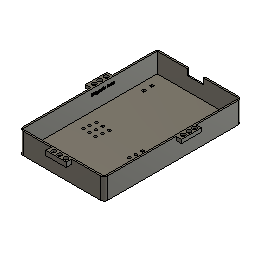
robot base (Autodesk Fusion 360 design; units mm, degrees)
Autodesk Fusion 360 part; units mm, degrees
(part 1 of 7)
sketch "Sketch1" plane through (0, 0, 0) normal (0, 1, 0) x (1, 0, 0)
  line L0 (-25, 75) -> (125, 75)
  line L1 (125, 75) -> (125, -175)
  line L2 (125, -175) -> (-25, -175)
  line L3 (-25, -175) -> (-25, 75)
  dimension "d1" = 150
  dimension "d2" = 250
  constraint horizontal L0
  constraint vertical L1
  constraint horizontal L2
  constraint vertical L3
  measures "d1" distance of L0.start L0.end
  measures "d2" distance of L0.start L2.end
extrude "Extrude1" add sketch "Sketch1" along normal blind 3 makes body 1
sketch "Sketch2" plane through (0, 3, 0) normal (0, 1, 0) x (-1, 0, 0)
  line L0 (25, 175) -> (-125, 175)
  line L1 (-125, 175) -> (-125, -75)
  line L2 (-125, -75) -> (25, -75)
  line L3 (25, -75) -> (25, 175)
sketch "Sketch3" plane through (0, 0, 0) normal (0, 1, 0) x (1, 0, 0)
  line L0 (-30, 80) -> (130, 80)
  line L1 (130, 80) -> (130, -180)
  line L2 (130, -180) -> (-30, -180)
  line L3 (-30, -180) -> (-30, 80)
  line L4 (-25, 75) -> (-25, -175)
  line L5 (125, -175) -> (125, 75)
  line L6 (125, 75) -> (-25, 75)
  dimension "d5" = 5
  dimension "d6" = 5
  dimension "d7" = 5
  constraint horizontal L0
  constraint vertical L1
  constraint horizontal L2
  constraint vertical L3
  measures "d5" distance of L3 L4
  measures "d6" distance of L1 L5
  measures "d7" distance of L0 L6
extrude "Extrude2" add sketch "Sketch3" along normal blind 40 bodies 1
shell "Shell1" thickness 3 removed faces 1 at (23.3333, 40, 93.3333) on bodies 1
move_body "Move1" bodies 1 to x (1, 0, 0) y (0, 1, 0) z (0, 0, 1) at (0, 60, 0)
sketch "Sketch4" plane through (0, 63, 0) normal (0, 1, 0) x (-1, 0, 0)
  line L0 (27, 177) -> (-127, 177)
  line L1 (-127, 177) -> (-127, -77)
  line L2 (-127, -77) -> (27, -77)
  line L3 (27, -77) -> (27, 177)
  line L4 (14.9226, -39.638) -> (9.9226, -39.638)
  line L5 (9.9226, -39.638) -> (9.9226, -34.638)
  line L6 (9.9226, -34.638) -> (14.9226, -34.638)
  line L7 (14.9226, -34.638) -> (14.9226, -39.638)
  line L8 (12.4226, 146.4275) -> (17.4226, 146.4275)
  line L9 (17.4226, 146.4275) -> (17.4226, 151.4275)
  line L10 (17.4226, 151.4275) -> (12.4226, 151.4275)
  line L11 (12.4226, 151.4275) -> (12.4226, 146.4275)
  line L12 (-110.5201, -34.638) -> (-105.5201, -34.638)
  line L13 (-105.5201, -34.638) -> (-105.5201, -39.638)
  line L14 (-105.5201, -39.638) -> (-110.5201, -39.638)
  line L15 (-110.5201, -39.638) -> (-110.5201, -34.638)
  line L16 (-105.5201, 145.9612) -> (-110.5201, 145.9612)
  line L17 (-110.5201, 145.9612) -> (-110.5201, 150.9612)
  line L18 (-110.5201, 150.9612) -> (-105.5201, 150.9612)
  line L19 (-105.5201, 150.9612) -> (-105.5201, 145.9612)
  dimension "d11" = 5
  dimension "d12" = 5
  dimension "d13" = 5
  dimension "d14" = 5
  dimension "d15" = 5
  dimension "d16" = 5
  dimension "d17" = 5
  dimension "d18" = 5
  constraint horizontal L4
  constraint vertical L5
  constraint horizontal L6
  constraint vertical L7
  constraint horizontal L8
  constraint vertical L9
  constraint horizontal L10
  constraint vertical L11
  constraint horizontal L12
  constraint vertical L13
  constraint horizontal L14
  constraint vertical L15
  constraint horizontal L16
  constraint vertical L17
  constraint horizontal L18
  constraint vertical L19
  measures "d11" distance of L4.start L4.end
  measures "d12" distance of L4.start L6.end
  measures "d13" distance of L8.start L8.end
  measures "d14" distance of L8.start L10.end
  measures "d15" distance of L12.start L12.end
  measures "d16" distance of L12.start L14.end
  measures "d17" distance of L16.start L16.end
  measures "d18" distance of L16.start L18.end
extrude "Extrude3" cut sketch "Sketch4" against normal blind 90 contours L4 L5 L6 L7 | L8 L9 L10 L11 | L12 L13 L14 L15 | L16 L17 L18 L19 bodies 1
sketch "Sketch5" plane through (0, 60, 0) normal (0, -1, 0) x (1, 0, 0)
  line L0 (110.5201, 150.9612) -> (110.5201, 145.9612)
  line L1 (110.5201, 145.9612) -> (105.5201, 145.9612)
  line L2 (105.5201, 145.9612) -> (105.5201, 150.9612)
  line L3 (105.5201, 150.9612) -> (110.5201, 150.9612)
  line L4 (105.5201, -39.638) -> (105.5201, -34.638)
  line L5 (105.5201, -34.638) -> (110.5201, -34.638)
  line L6 (110.5201, -34.638) -> (110.5201, -39.638)
  line L7 (110.5201, -39.638) -> (105.5201, -39.638)
  line L8 (-12.4226, 146.4275) -> (-17.4226, 146.4275)
  line L9 (-17.4226, 146.4275) -> (-17.4226, 151.4275)
  line L10 (-17.4226, 151.4275) -> (-12.4226, 151.4275)
  line L11 (-12.4226, 151.4275) -> (-12.4226, 146.4275)
  line L12 (-9.9226, -34.638) -> (-9.9226, -39.638)
  line L13 (-9.9226, -39.638) -> (-14.9226, -39.638)
  line L14 (-14.9226, -39.638) -> (-14.9226, -34.638)
  line L15 (-14.9226, -34.638) -> (-9.9226, -34.638)
  line L16 (130, 180) -> (-30, 180)
  line L17 (-30, 180) -> (-30, -80)
  line L18 (-30, -80) -> (130, -80)
  line L19 (130, -80) -> (130, 180)
  line L20 (-24.7646, 143.5608) -> (-4.7646, 143.5608)
  line L21 (-4.7646, 143.5608) -> (-4.7646, 93.5608)
  line L22 (-4.7646, 93.5608) -> (-24.7646, 93.5608)
  line L23 (-24.7646, 93.5608) -> (-24.7646, 143.5608)
  line L24 (-24.5171, 4.1257) -> (-4.5171, 4.1257)
  line L25 (-4.5171, 4.1257) -> (-4.5171, -45.8743)
  line L26 (-4.5171, -45.8743) -> (-24.5171, -45.8743)
  line L27 (-24.5171, -45.8743) -> (-24.5171, 4.1257)
  line L28 (123.4565, -45.8596) -> (103.4565, -45.8596)
  line L29 (103.4565, -45.8596) -> (103.4565, 4.1404)
  line L30 (103.4565, 4.1404) -> (123.4565, 4.1404)
  line L31 (123.4565, 4.1404) -> (123.4565, -45.8596)
  line L32 (104.6989, 143.7931) -> (124.6989, 143.7931)
  line L33 (124.6989, 143.7931) -> (124.6989, 93.7931)
  line L34 (124.6989, 93.7931) -> (104.6989, 93.7931)
  line L35 (104.6989, 93.7931) -> (104.6989, 143.7931)
  dimension "d21" = 20
  dimension "d22" = 50
  dimension "d23" = 20
  dimension "d24" = 50
  dimension "d25" = 20
  dimension "d26" = 50
  dimension "d27" = 20
  dimension "d28" = 50
  constraint horizontal L20
  constraint vertical L21
  constraint horizontal L22
  constraint vertical L23
  constraint horizontal L24
  constraint vertical L25
  constraint horizontal L26
  constraint vertical L27
  constraint horizontal L28
  constraint vertical L29
  constraint horizontal L30
  constraint vertical L31
  constraint horizontal L32
  constraint horizontal L34
  constraint vertical L35
  measures "d21" distance of L20.start L20.end
  measures "d22" distance of L20.start L22.end
  measures "d23" distance of L24.start L24.end
  measures "d24" distance of L24.start L26.end
  measures "d25" distance of L28.start L28.end
  measures "d26" distance of L28.start L30.end
  measures "d27" distance of L32.start L32.end
  measures "d28" distance of L32.start L34.end
extrude "Extrude4" add sketch "Sketch5" along normal blind 2 contours L4 L5 L6 L7 | L12 L13 L14 L15 | L20 L21 L22 L23 | L24 L25 L26 L27 | L28 L29 L30 L31 | L32 L33 L34 L35 bodies 1
sketch "Sketch6" plane through (0, 0, 0) normal (0, 1, 0) x (1, 0, 0)
  line L0 (-200, 100) -> (-40, 100)
  line L1 (-40, 100) -> (-40, -155)
  line L2 (-40, -155) -> (-200, -155)
  line L3 (-200, -155) -> (-200, 100)
  dimension "d31" = 160
  dimension "d32" = 255
  constraint horizontal L0
  constraint vertical L1
  constraint horizontal L2
  constraint vertical L3
  measures "d31" distance of L0.start L0.end
  measures "d32" distance of L0.start L2.end
sketch "Sketch7" plane through (0, 49.0351, -11.7723) normal (0, 0.97237, -0.233445) x (-1, 0, 0)
  line L0 (210, -96.898) -> (210, 166.4916)
  line L1 (210, 166.4916) -> (50, 166.4916)
  line L2 (50, 166.4916) -> (50, -96.898)
  line L3 (107.3171, 129.6816) -> (144.3171, 129.6816)
  line L4 (144.3171, 129.6816) -> (144.3171, 100.6816)
  line L5 (144.3171, 100.6816) -> (107.3171, 100.6816)
  line L6 (107.3171, 100.6816) -> (107.3171, 129.6816)
  line L7 (50, -96.898) -> (210, -96.898)
  dimension "d38" = 37
  dimension "d39" = 29
  constraint horizontal L3
  constraint vertical L4
  constraint horizontal L5
  constraint vertical L6
  measures "d38" distance of L3.start L3.end
  measures "d39" distance of L3.start L5.end
sketch "Sketch8" plane through (0, 49.0351, -11.7723) normal (0, 0.97237, -0.233445) x (-1, 0, 0)
  line L0 (144.3171, 129.6816) -> (144.3171, 100.6816)
  line L1 (144.3171, 100.6816) -> (107.3171, 100.6816)
  line L2 (107.3171, 100.6816) -> (107.3171, 129.6816)
  line L3 (107.3171, 129.6816) -> (144.3171, 129.6816)
  line L4 (210, -96.898) -> (210, 166.4916)
  line L5 (210, 166.4916) -> (50, 166.4916)
  line L6 (50, 166.4916) -> (50, -96.898)
  line L7 (50, -96.898) -> (210, -96.898)
copy_body "Body->Comp2" bodies 1 removing the originals makes body 2 in component "base"
sketch "Sketch9" plane through (0, 100, 0) normal (0, 1, 0) x (-1, 0, 0)
  line L0 (27, 177) -> (27, -77)
  line L1 (27, -77) -> (-127, -77)
  line L2 (-127, -77) -> (-127, 177)
  line L3 (-127, 177) -> (27, 177)
  line L4 (30, 180) -> (-130, 180)
  line L5 (-130, 180) -> (-130, -80)
  line L6 (-130, -80) -> (30, -80)
  line L7 (30, -80) -> (30, 180)
sketch "Sketch10" plane through (-30, 0, 0) normal (-1, 0, 0) x (0, 0, 1)
  line L0 (-80, 60) -> (180, 60)
  line L1 (180, 60) -> (180, 100)
  line L2 (180, 100) -> (-80, 100)
  line L3 (-80, 100) -> (-80, 60)
  line L4 (5, 100) -> (45, 100)
  line L5 (45, 100) -> (45, 94.0332)
  line L6 (45, 94.0332) -> (5, 94.0332)
  line L7 (5, 94.0332) -> (5, 100)
  dimension "d46" = 40
  constraint horizontal L4
  constraint vertical L5
  constraint horizontal L6
  constraint vertical L7
  constraint coincident L2 L4.start
  measures "d46" distance of L4.start L4.end
extrude "Extrude1'" add sketch "Sketch10" along normal blind 10 contours L2 L4 L5 L6 L7 bodies 2 in component "base"
sketch "Sketch11" plane through (0, 100, 0) normal (0, 1, 0) x (-1, 0, 0)
  line L0 (27, 177) -> (27, -77)
  line L1 (27, -77) -> (-127, -77)
  line L2 (-127, -77) -> (-127, 177)
  line L3 (-127, 177) -> (27, 177)
  line L4 (30, 180) -> (-130, 180)
  line L5 (-130, 180) -> (-130, -80)
  line L6 (-130, -80) -> (30, -80)
  line L7 (30, -80) -> (30, 5)
  line L8 (30, 5) -> (40, 5)
  line L9 (40, 5) -> (40, 45)
  line L10 (40, 45) -> (30, 45)
  line L11 (30, 45) -> (30, 180)
  circle A0 centre (33.1089, 35.6235) radius 4
  circle A1 centre (33.528, 24.7269) radius 4
  circle A2 centre (33.7376, 12.573) radius 4
  dimension "d49" = 8
  dimension "d50" = 8
  dimension "d51" = 8
  measures "d49" diameter of A0
  measures "d50" diameter of A1
  measures "d51" diameter of A2
extrude "Extrude2'" cut sketch "Sketch11" against normal blind 4 contours A0 | A1 | A2 bodies 2 in component "base"
sketch "Sketch12" plane through (130, 0, 0) normal (1, 0, 0) x (0, 0, -1)
  line L0 (-180, 60) -> (80, 60)
  line L1 (80, 60) -> (80, 100)
  line L2 (80, 100) -> (-180, 100)
  line L3 (-180, 100) -> (-180, 60)
  line L4 (-44.1105, 100) -> (-6.5994, 100)
  line L5 (-6.5994, 100) -> (-6.5994, 93.0994)
  line L6 (-6.5994, 93.0994) -> (-44.1105, 93.0994)
  line L7 (-44.1105, 93.0994) -> (-44.1105, 100)
  constraint horizontal L4
  constraint horizontal L6
  constraint vertical L7
  constraint coincident L2 L4.start
extrude "Extrude3'" add sketch "Sketch12" along normal blind 10 contours L2 L4 L5 L6 L7 bodies 2 in component "base"
sketch "Sketch13" plane through (0, 100, 0) normal (0, 1, 0) x (-1, 0, 0)
  circle A0 centre (33.1089, 35.6235) radius 4
  circle A1 centre (33.528, 24.7269) radius 4
  circle A2 centre (33.7376, 12.573) radius 4
  line L0 (27, 177) -> (27, -77)
  line L1 (27, -77) -> (-127, -77)
  line L2 (-127, -77) -> (-127, 177)
  line L3 (-127, 177) -> (27, 177)
  line L4 (30, 180) -> (-130, 180)
  line L5 (-130, 180) -> (-130, 44.1105)
  line L6 (-130, 44.1105) -> (-140, 44.1105)
  line L7 (-140, 44.1105) -> (-140, 6.5994)
  line L8 (-140, 6.5994) -> (-130, 6.5994)
  line L9 (-130, 6.5994) -> (-130, -80)
  line L10 (-130, -80) -> (30, -80)
  line L11 (30, -80) -> (30, 5)
  line L12 (30, 5) -> (40, 5)
  line L13 (40, 5) -> (40, 45)
  line L14 (40, 45) -> (30, 45)
  line L15 (30, 45) -> (30, 180)
sketch "Sketch14" plane through (130, 0, 0) normal (1, 0, 0) x (0, 0, -1)
sketch "Sketch15" plane through (0, 100, 0) normal (0, 1, 0) x (-1, 0, 0)
  circle A0 centre (-133.6931, 13.6208) radius 4
  circle A1 centre (-134, 24) radius 4
  circle A2 centre (-134, 35) radius 4
  dimension "d56" = 8
  dimension "d57" = 8
  dimension "d58" = 8
  measures "d56" diameter of A0
  measures "d57" diameter of A1
  measures "d58" diameter of A2
extrude "Extrude4'" cut sketch "Sketch15" against normal blind 4 bodies 2 in component "base"
sketch "Sketch16" plane through (131.259, 0, 0) normal (1, 0, 0) x (0, 0, -1)
  line L0 (-178.8896, 102.3306) -> (76.1007, 100.1054)
  line L1 (76.1007, 100.1054) -> (76.136, 104.1577)
  line L2 (76.136, 104.1577) -> (-178.2788, 172.328)
  line L3 (-178.2788, 172.328) -> (-178.8896, 102.3306)
  line L4 (-45, 110) -> (-6.7003, 110)
  line L5 (-6.7003, 110) -> (-6.7003, 101.218)
  line L6 (-6.7003, 101.218) -> (-45, 101.218)
  line L7 (-45, 101.218) -> (-45, 110)
  constraint horizontal L4
  constraint vertical L5
  constraint horizontal L6
  constraint vertical L7
sketch "Sketch17" plane through (0, 100, 0) normal (0, 1, 0) x (-1, 0, 0)
  circle A0 centre (-136.21, 34.8) radius 4
  circle A1 centre (-135.94, 25.4) radius 4
  circle A2 centre (-135.73, 15.73) radius 4
  dimension "d63" = 8
  dimension "d64" = 8
  dimension "d65" = 8
  measures "d63" diameter of A0
  measures "d64" diameter of A1
  measures "d65" diameter of A2
sketch "Sketch18" plane through (-29.741, 0, 0) normal (-1, 0, 0) x (0, 0, 1)
  line L0 (-76.1007, 100.1054) -> (178.8896, 102.3306)
  line L1 (178.8896, 102.3306) -> (178.2788, 172.328)
  line L2 (178.2788, 172.328) -> (-76.136, 104.1577)
  line L3 (-76.136, 104.1577) -> (-76.1007, 100.1054)
  line L4 (4.8558, 101.218) -> (45, 101.218)
  line L5 (45, 101.218) -> (45, 108)
  line L6 (45, 108) -> (4.8558, 108)
  line L7 (4.8558, 108) -> (4.8558, 101.218)
  constraint horizontal L4
  constraint vertical L5
  constraint horizontal L6
  constraint vertical L7
sketch "Sketch19" plane through (0, 101.218, 0) normal (0, -1, 0) x (1, 0, 0)
  line L0 (-29.741, 4.8558) -> (-29.741, 45)
  line L1 (-29.741, 45) -> (-39.741, 45)
  line L2 (-39.741, 45) -> (-39.741, 4.8558)
  line L3 (-39.741, 4.8558) -> (-29.741, 4.8558)
  circle A0 centre (-35, 13) radius 4
  circle A1 centre (-35, 23) radius 4
  circle A2 centre (-35, 33) radius 4
  dimension "d70" = 8
  dimension "d71" = 8
  dimension "d72" = 8
  measures "d70" diameter of A0
  measures "d71" diameter of A1
  measures "d72" diameter of A2
sketch "Sketch20" plane through (0, 0, 180) normal (0, 0, 1) x (1, 0, 0)
  line L0 (-30, 60) -> (130, 60)
  line L1 (130, 60) -> (130, 100)
  line L2 (130, 100) -> (-30, 100)
  line L3 (-30, 100) -> (-30, 60)
  line L4 (30, 100) -> (68.2649, 100)
  line L5 (68.2649, 100) -> (68.2649, 91.3001)
  line L6 (68.2649, 91.3001) -> (30, 91.3001)
  line L7 (30, 91.3001) -> (30, 100)
  constraint horizontal L4
  constraint vertical L5
  constraint horizontal L6
  constraint vertical L7
  constraint coincident L2 L4.start
extrude "Extrude5" add sketch "Sketch20" along normal blind 10 contours L2 L4 L5 L6 L7 bodies 2 in component "base"
sketch "Sketch21" plane through (0, 0, 0) normal (0, 0, 1) x (1, 0, 0)
sketch "Sketch22" plane through (0, 100, 0) normal (0, 1, 0) x (-1, 0, 0)
  circle A0 centre (-134, 35) radius 4
  circle A1 centre (-134, 24) radius 4
  circle A2 centre (-133.6931, 13.6208) radius 4
  circle A3 centre (33.1089, 35.6235) radius 4
  circle A4 centre (33.528, 24.7269) radius 4
  circle A5 centre (33.7376, 12.573) radius 4
  line L0 (27, 177) -> (27, -77)
  line L1 (27, -77) -> (-127, -77)
  line L2 (-127, -77) -> (-127, 177)
  line L3 (-127, 177) -> (27, 177)
  line L4 (30, 180) -> (-30, 180)
  line L5 (-30, 180) -> (-30, 190)
  line L6 (-30, 190) -> (-68.2649, 190)
  line L7 (-68.2649, 190) -> (-68.2649, 180)
  line L8 (-68.2649, 180) -> (-130, 180)
  line L9 (-130, 180) -> (-130, 44.1105)
  line L10 (-130, 44.1105) -> (-140, 44.1105)
  line L11 (-140, 44.1105) -> (-140, 6.5994)
  line L12 (-140, 6.5994) -> (-130, 6.5994)
  line L13 (-130, 6.5994) -> (-130, -80)
  line L14 (-130, -80) -> (30, -80)
  line L15 (30, -80) -> (30, 5)
  line L16 (30, 5) -> (40, 5)
  line L17 (40, 5) -> (40, 45)
  line L18 (40, 45) -> (30, 45)
  line L19 (30, 45) -> (30, 180)
  circle A6 centre (-39, 184) radius 4
  circle A7 centre (-50, 184) radius 4
  circle A8 centre (-62, 184) radius 4
  dimension "d77" = 8
  dimension "d78" = 8
  dimension "d79" = 8
  measures "d77" diameter of A6
  measures "d78" diameter of A7
  measures "d79" diameter of A8
extrude "Extrude6" cut sketch "Sketch22" against normal blind 4 contours A6 | A7 | A8 bodies 2 in component "base"
sketch "Sketch23" plane through (0, 1.5688, 179.7689) normal (0, 0.008727, 0.999962) x (1, 0, 0)
  line L0 (-29.741, 100.7657) -> (130.259, 100.7657)
  line L1 (130.259, 100.7657) -> (130.259, 170.7657)
  line L2 (130.259, 170.7657) -> (-29.741, 170.7657)
  line L3 (-29.741, 170.7657) -> (-29.741, 100.7657)
  line L4 (30, 109) -> (68.1162, 109)
  line L5 (68.1162, 109) -> (68.1162, 100.7657)
  line L6 (68.1162, 100.7657) -> (30, 100.7657)
  line L7 (30, 100.7657) -> (30, 109)
  constraint horizontal L4
  constraint horizontal L6
  constraint vertical L7
  constraint coincident L0 L5.end
sketch "Sketch24" plane through (0, 100.7618, -0.8793) normal (0, -0.999962, 0.008727) x (1, 0, 0)
  line L0 (127.259, 176.7758) -> (127.259, -72.2242)
  line L1 (127.259, -72.2242) -> (-26.741, -72.2242)
  line L2 (-26.741, -72.2242) -> (-26.741, 176.7758)
  line L3 (-26.741, 176.7758) -> (127.259, 176.7758)
  line L4 (-29.741, -75.2242) -> (130.259, -75.2242)
  line L5 (130.259, -75.2242) -> (130.259, 179.7758)
  line L6 (130.259, 179.7758) -> (68.1162, 179.7758)
  line L7 (68.1162, 179.7758) -> (68.1162, 190.7758)
  line L8 (68.1162, 190.7758) -> (30, 190.7758)
  line L9 (30, 190.7758) -> (30, 179.7758)
  line L10 (30, 179.7758) -> (-29.741, 179.7758)
  line L11 (-29.741, 179.7758) -> (-29.741, -75.2242)
  circle A0 centre (39.3165, 184.6097) radius 4
  circle A1 centre (50, 185) radius 4
  circle A2 centre (60, 185) radius 4
  dimension "d84" = 8
  dimension "d85" = 8
  dimension "d86" = 8
  measures "d84" diameter of A0
  measures "d85" diameter of A1
  measures "d86" diameter of A2
sketch "Sketch25" plane through (0, 1.5688, 179.7689) normal (0, 0.008727, 0.999962) x (1, 0, 0)
  line L0 (68.1162, 109) -> (68.1162, 100.7657)
  line L1 (68.1162, 100.7657) -> (130.259, 100.7657)
  line L2 (130.259, 100.7657) -> (130.259, 170.7657)
  line L3 (130.259, 170.7657) -> (-29.741, 170.7657)
  line L4 (-29.741, 170.7657) -> (-29.741, 100.7657)
  line L5 (-29.741, 100.7657) -> (30, 100.7657)
  line L6 (30, 100.7657) -> (30, 109)
  line L7 (30, 109) -> (68.1162, 109)
  line L8 (5, 145) -> (10, 145)
  line L9 (10, 145) -> (10, 135)
  line L10 (10, 135) -> (5, 135)
  line L11 (5, 135) -> (5, 145)
  line L12 (15, 145) -> (20, 145)
  line L13 (20, 145) -> (20, 135)
  line L14 (20, 135) -> (15, 135)
  line L15 (15, 135) -> (15, 145)
  line L16 (25, 145) -> (30, 145)
  line L17 (30, 145) -> (30, 135)
  line L18 (30, 135) -> (25, 135)
  line L19 (25, 135) -> (25, 145)
  line L20 (35, 145) -> (40, 145)
  line L21 (40, 145) -> (40, 135)
  line L22 (40, 135) -> (35, 135)
  line L23 (35, 135) -> (35, 145)
  line L24 (45, 145) -> (50, 145)
  line L25 (50, 145) -> (50, 135)
  line L26 (50, 135) -> (45, 135)
  line L27 (45, 135) -> (45, 145)
  line L28 (55, 145) -> (60, 145)
  line L29 (60, 145) -> (60, 135)
  line L30 (60, 135) -> (55, 135)
  line L31 (55, 135) -> (55, 145)
  line L32 (65, 145) -> (70, 145)
  line L33 (70, 145) -> (70, 135)
  line L34 (70, 135) -> (65, 135)
  line L35 (65, 135) -> (65, 145)
  line L36 (75, 145) -> (80, 145)
  line L37 (80, 145) -> (80, 135)
  line L38 (80, 135) -> (75, 135)
  line L39 (75, 135) -> (75, 145)
  line L40 (85, 145) -> (90, 145)
  line L41 (90, 145) -> (90, 135)
  line L42 (90, 135) -> (85, 135)
  line L43 (85, 135) -> (85, 145)
  line L44 (95, 145) -> (100, 145)
  line L45 (100, 145) -> (100, 135)
  line L46 (100, 135) -> (95, 135)
  line L47 (95, 135) -> (95, 145)
  line L48 (5, 125) -> (10, 125)
  line L49 (10, 125) -> (10, 115)
  line L50 (10, 115) -> (5, 115)
  line L51 (5, 115) -> (5, 125)
  line L52 (15, 125) -> (20, 125)
  line L53 (20, 125) -> (20, 115)
  line L54 (20, 115) -> (15, 115)
  line L55 (15, 115) -> (15, 125)
  line L56 (25, 125) -> (30, 125)
  line L57 (30, 125) -> (30, 115)
  line L58 (30, 115) -> (25, 115)
  line L59 (25, 115) -> (25, 125)
  line L60 (35, 125) -> (40, 125)
  line L61 (40, 125) -> (40, 115)
  line L62 (40, 115) -> (35, 115)
  line L63 (35, 115) -> (35, 125)
  line L64 (45, 125) -> (50, 125)
  line L65 (50, 125) -> (50, 115)
  line L66 (50, 115) -> (45, 115)
  line L67 (45, 115) -> (45, 125)
  line L68 (55, 125) -> (60, 125)
  line L69 (60, 125) -> (60, 115)
  line L70 (60, 115) -> (55, 115)
  line L71 (55, 115) -> (55, 125)
  line L72 (65, 125) -> (70, 125)
  line L73 (70, 125) -> (70, 115)
  line L74 (70, 115) -> (65, 115)
  line L75 (65, 115) -> (65, 125)
  line L76 (75, 125) -> (80, 125)
  line L77 (80, 125) -> (80, 115)
  line L78 (80, 115) -> (75, 115)
  line L79 (75, 115) -> (75, 125)
  line L80 (85, 125) -> (90, 125)
  line L81 (90, 125) -> (90, 115)
  line L82 (90, 115) -> (85, 115)
  line L83 (85, 115) -> (85, 125)
  line L84 (95, 125) -> (100, 125)
  line L85 (100, 125) -> (100, 115)
  line L86 (100, 115) -> (95, 115)
  line L87 (95, 115) -> (95, 125)
  constraint horizontal L8
  constraint vertical L9
  constraint horizontal L10
  constraint vertical L11
  constraint horizontal L12
  constraint vertical L13
  constraint horizontal L14
  constraint vertical L15
  constraint horizontal L16
  constraint vertical L17
  constraint horizontal L18
  constraint vertical L19
  constraint horizontal L20
  constraint vertical L21
  constraint horizontal L22
  constraint vertical L23
  constraint horizontal L24
  constraint vertical L25
  constraint horizontal L26
  constraint vertical L27
  constraint horizontal L28
  constraint vertical L29
  constraint horizontal L30
  constraint vertical L31
  constraint horizontal L32
  constraint vertical L33
  constraint horizontal L34
  constraint vertical L35
  constraint horizontal L36
  constraint vertical L37
  constraint horizontal L38
  constraint vertical L39
  constraint horizontal L40
  constraint vertical L41
  constraint horizontal L42
  constraint vertical L43
  constraint horizontal L44
  constraint vertical L45
  constraint horizontal L46
  constraint vertical L47
  constraint horizontal L48
  constraint vertical L49
  constraint horizontal L50
  constraint vertical L51
  constraint horizontal L52
  constraint vertical L53
  constraint horizontal L54
  constraint vertical L55
  constraint horizontal L56
  constraint vertical L57
  constraint horizontal L58
  constraint vertical L59
  constraint horizontal L60
  constraint vertical L61
  constraint horizontal L62
  constraint vertical L63
  constraint horizontal L64
  constraint vertical L65
  constraint horizontal L66
  constraint vertical L67
  constraint horizontal L68
  constraint vertical L69
  constraint horizontal L70
  constraint vertical L71
  constraint horizontal L72
  constraint vertical L73
  constraint horizontal L74
  constraint vertical L75
  constraint horizontal L76
  constraint vertical L77
  constraint horizontal L78
  constraint vertical L79
  constraint horizontal L80
  constraint vertical L81
  constraint horizontal L82
  constraint vertical L83
  constraint horizontal L84
  constraint vertical L85
  constraint horizontal L86
  constraint vertical L87
sketch "Sketch26" plane through (-29.741, 0, 0) normal (-1, 0, 0) x (0, 0, 1)
  line L0 (4.8558, 108) -> (45, 108)
  line L1 (45, 108) -> (45, 101.218)
  line L2 (45, 101.218) -> (4.8558, 101.218)
  line L3 (4.8558, 101.218) -> (4.8558, 108)
  line L4 (-76.1007, 100.1054) -> (178.8896, 102.3306)
  line L5 (178.8896, 102.3306) -> (178.2788, 172.328)
  line L6 (178.2788, 172.328) -> (-76.136, 104.1577)
  line L7 (-76.136, 104.1577) -> (-76.1007, 100.1054)
sketch "Sketch27" plane through (0, 63, 0) normal (0, 1, 0) x (-1, 0, 0)
  line L0 (-110.5201, 145.9612) -> (-110.5201, 150.9612)
  line L1 (-110.5201, 150.9612) -> (-105.5201, 150.9612)
  line L2 (-105.5201, 150.9612) -> (-105.5201, 145.9612)
  line L3 (-105.5201, 145.9612) -> (-110.5201, 145.9612)
  line L4 (-105.5201, -34.638) -> (-105.5201, -39.638)
  line L5 (-105.5201, -39.638) -> (-110.5201, -39.638)
  line L6 (-110.5201, -39.638) -> (-110.5201, -34.638)
  line L7 (-110.5201, -34.638) -> (-105.5201, -34.638)
  line L8 (17.4226, 146.4275) -> (12.4226, 146.4275)
  line L9 (12.4226, 146.4275) -> (12.4226, 151.4275)
  line L10 (12.4226, 151.4275) -> (17.4226, 151.4275)
  line L11 (17.4226, 151.4275) -> (17.4226, 146.4275)
  line L12 (9.9226, -39.638) -> (9.9226, -34.638)
  line L13 (9.9226, -34.638) -> (14.9226, -34.638)
  line L14 (14.9226, -34.638) -> (14.9226, -39.638)
  line L15 (14.9226, -39.638) -> (9.9226, -39.638)
  line L16 (27, 177) -> (-127, 177)
  line L17 (-127, 177) -> (-127, -77)
  line L18 (-127, -77) -> (27, -77)
  line L19 (27, -77) -> (27, 177)
  line L20 (-106.0146, 110.336) -> (-106.0146, 147.3829) construction
  line L21 (-106.0146, 147.3829) -> (-117.9945, 147.3829) construction
  line L22 (-117.9945, 147.3829) -> (-117.9945, 110.336) construction
  line L23 (-117.9945, 110.336) -> (-106.0146, 110.336) construction
  dimension "d91" = 6
  text T0 "Hole for\nTT wire" font "Arial" height 6 align left top in box 37.0468 x 11.9799 at (-106.0146, 110.336) x (0, 1) y (-1, 0) spacing 1 kerned
sketch "Sketch28" plane through (0, 0, 0) normal (0, 0, 1) x (1, 0, 0)
sketch "Sketch29" plane through (0, 0, 0) normal (0, 0, 1) x (1, 0, 0)
extrude "Extrude7" cut sketch "Sketch27" against normal blind 1.5 text T0 bodies 2 in component "base"
sketch "Sketch30" plane through (0, 0, 177) normal (0, 0, -1) x (-1, 0, 0)
  line L0 (-127, 63) -> (27, 63)
  line L1 (27, 63) -> (27, 100)
  line L2 (27, 100) -> (-127, 100)
  line L3 (-127, 100) -> (-127, 63)
  line L4 (-82.8733, 77.686) -> (-13.3336, 77.0675) construction
  line L5 (-13.3336, 77.0675) -> (-13.2091, 91.0673) construction
  line L6 (-13.2091, 91.0673) -> (-82.7488, 91.6857) construction
  line L7 (-82.7488, 91.6857) -> (-82.8733, 77.686) construction
  dimension "d95" = 6
  dimension "d96" = 0
  text T0 "Gethin Robot v1" font "Arial" height 6 bold align left top in box 69.5425 x 14.0003 at (-82.8733, 77.686) x (0.99996, -0.008893) y (0.008893, 0.99996) spacing 1 kerned
extrude "Extrude8" cut sketch "Sketch30" against normal blind 1.5 text T0 bodies 2 in component "base"
sketch "Sketch31" plane through (-27, 0, 0) normal (1, 0, 0) x (0, 0, -1)
  line L0 (-177, 63) -> (77, 63)
  line L1 (77, 63) -> (77, 100)
  line L2 (77, 100) -> (-177, 100)
  line L3 (-177, 100) -> (-177, 63)
  line L4 (-46.978, 84.5868) -> (2.0388, 84.3472) construction
  line L5 (2.0388, 84.3472) -> (2.0772, 92.1978) construction
  line L6 (2.0772, 92.1978) -> (-46.9396, 92.4374) construction
  line L7 (-46.9396, 92.4374) -> (-46.978, 84.5868) construction
  dimension "d99" = 5
  text T0 "Magnets here" font "Arial" height 5 bold align left top in box 49.0173 x 7.8507 at (-46.978, 84.5868) x (0.999988, -0.004888) y (0.004888, 0.999988) spacing 1 kerned
extrude "Extrude9" cut sketch "Sketch31" against normal blind 1.5 text T0 bodies 2 in component "base"
fillet "Fillet1" radius 7 2 edges at (-30, 80, 180) (130, 80, 180) on bodies 2 in component "base"
fillet "Fillet2" radius 7 1 edges at (130, 80, -80) on bodies 2 in component "base"
fillet "Fillet3" radius 7 1 edges at (-30, 80, -80) on bodies 2 in component "base"
sketch "Sketch32" plane through (0, 116.2145, -31.1396) normal (0, 0.965926, -0.258819) x (-1, 0, 0)
  ellipse E0 centre (22.741, -39.3535) end of major axis (22.741, -46.5838) minor radius 7 (22.741, -46.5838) -> (29.741, -39.3535) ccw
  line L0 (29.741, -39.3535) -> (29.741, 209.5755)
  ellipse E1 centre (22.741, 209.5755) end of major axis (22.741, 216.8058) minor radius 7 (29.741, 209.5755) -> (22.741, 216.8058) ccw
  line L1 (22.741, 216.8058) -> (-123.259, 216.8058)
  ellipse E2 centre (-123.259, 209.5755) end of major axis (-123.259, 216.8058) minor radius 7 (-123.259, 216.8058) -> (-130.259, 209.5755) ccw
  line L2 (-130.259, 209.5755) -> (-130.259, -39.3535)
  ellipse E3 centre (-123.259, -39.3535) end of major axis (-123.259, -46.5838) minor radius 7 (-130.259, -39.3535) -> (-123.259, -46.5838) ccw
  line L3 (-123.259, -46.5838) -> (22.741, -46.5838)
  line L4 (-35.9419, 179.9959) -> (-35.9419, 150.9959)
  line L5 (-35.9419, 150.9959) -> (-72.9419, 150.9959)
  line L6 (-72.9419, 150.9959) -> (-72.9419, 179.9959)
  line L7 (-72.9419, 179.9959) -> (-35.9419, 179.9959)
sketch "Sketch33" plane through (0, 116.2145, -31.1396) normal (0, 0.965926, -0.258819) x (-1, 0, 0)
  ellipse E0 centre (22.741, -39.3535) end of major axis (22.741, -46.5838) minor radius 7 (22.741, -46.5838) -> (29.741, -39.3535) ccw
  line L0 (29.741, -39.3535) -> (29.741, 209.5755)
  ellipse E1 centre (22.741, 209.5755) end of major axis (22.741, 216.8058) minor radius 7 (29.741, 209.5755) -> (22.741, 216.8058) ccw
  line L1 (22.741, 216.8058) -> (-123.259, 216.8058)
  ellipse E2 centre (-123.259, 209.5755) end of major axis (-123.259, 216.8058) minor radius 7 (-123.259, 216.8058) -> (-130.259, 209.5755) ccw
  line L2 (-130.259, 209.5755) -> (-130.259, -39.3535)
  ellipse E3 centre (-123.259, -39.3535) end of major axis (-123.259, -46.5838) minor radius 7 (-130.259, -39.3535) -> (-123.259, -46.5838) ccw
  line L3 (-123.259, -46.5838) -> (22.741, -46.5838)
  line L4 (-35.9419, 179.9959) -> (-35.9419, 150.9959)
  line L5 (-35.9419, 150.9959) -> (-72.9419, 150.9959)
  line L6 (-72.9419, 150.9959) -> (-72.9419, 179.9959)
  line L7 (-72.9419, 179.9959) -> (-35.9419, 179.9959)
sketch "Sketch34" plane through (0, 49.0351, -11.7723) normal (0, 0.97237, -0.233445) x (-1, 0, 0)
sketch "Sketch35" plane through (0, 116.2145, -31.1396) normal (0, 0.965926, -0.258819) x (-1, 0, 0)
  ellipse E0 centre (22.741, -39.3535) end of major axis (22.741, -46.5838) minor radius 7 (22.741, -46.5838) -> (29.741, -39.3535) ccw
  line L0 (29.741, -39.3535) -> (29.741, 209.5755)
  ellipse E1 centre (22.741, 209.5755) end of major axis (22.741, 216.8058) minor radius 7 (29.741, 209.5755) -> (22.741, 216.8058) ccw
  line L1 (22.741, 216.8058) -> (-123.259, 216.8058)
  ellipse E2 centre (-123.259, 209.5755) end of major axis (-123.259, 216.8058) minor radius 7 (-123.259, 216.8058) -> (-130.259, 209.5755) ccw
  line L2 (-130.259, 209.5755) -> (-130.259, -39.3535)
  ellipse E3 centre (-123.259, -39.3535) end of major axis (-123.259, -46.5838) minor radius 7 (-130.259, -39.3535) -> (-123.259, -46.5838) ccw
  line L3 (-123.259, -46.5838) -> (22.741, -46.5838)
  line L4 (-35.9419, 179.9959) -> (-35.9419, 150.9959)
  line L5 (-35.9419, 150.9959) -> (-72.9419, 150.9959)
  line L6 (-72.9419, 150.9959) -> (-72.9419, 179.9959)
  line L7 (-72.9419, 179.9959) -> (-35.9419, 179.9959)
sketch "Sketch36" plane through (0, 116.2145, -31.1396) normal (0, 0.965926, -0.258819) x (-1, 0, 0)
  ellipse E0 centre (22.741, -39.3535) end of major axis (22.741, -46.5838) minor radius 7 (22.741, -46.5838) -> (29.741, -39.3535) ccw
  line L0 (29.741, -39.3535) -> (29.741, 209.5755)
  ellipse E1 centre (22.741, 209.5755) end of major axis (22.741, 216.8058) minor radius 7 (29.741, 209.5755) -> (22.741, 216.8058) ccw
  line L1 (22.741, 216.8058) -> (-123.259, 216.8058)
  ellipse E2 centre (-123.259, 209.5755) end of major axis (-123.259, 216.8058) minor radius 7 (-123.259, 216.8058) -> (-130.259, 209.5755) ccw
  line L2 (-130.259, 209.5755) -> (-130.259, -39.3535)
  ellipse E3 centre (-123.259, -39.3535) end of major axis (-123.259, -46.5838) minor radius 7 (-130.259, -39.3535) -> (-123.259, -46.5838) ccw
  line L3 (-123.259, -46.5838) -> (22.741, -46.5838)
  line L4 (-35.9419, 179.9959) -> (-35.9419, 150.9959)
  line L5 (-35.9419, 150.9959) -> (-72.9419, 150.9959)
  line L6 (-72.9419, 150.9959) -> (-72.9419, 179.9959)
  line L7 (-72.9419, 179.9959) -> (-35.9419, 179.9959)
  line L8 (-105, 20) -> (4.5871, 20)
  line L9 (19.5871, 5) -> (19.5871, -24.3535)
  line L10 (4.5871, -39.3535) -> (-105, -39.3535)
  line L11 (-120, -24.3535) -> (-120, 5)
  arc A0 (-105, 20) -> (-120, 5) centre (-105, 5) ccw
  arc A1 (19.5871, 5) -> (4.5871, 20) centre (4.5871, 5) ccw
  arc A2 (4.5871, -39.3535) -> (19.5871, -24.3535) centre (4.5871, -24.3535) ccw
  arc A3 (-120, -24.3535) -> (-105, -39.3535) centre (-105, -24.3535) ccw
  dimension "d115" = 15
  constraint horizontal L8
  constraint vertical L9
  constraint horizontal L10
  constraint vertical L11
  constraint tangent L8 A0
  constraint tangent L11 A0
  constraint tangent L8 A1
  constraint tangent L9 A1
  constraint equal A0 A1
  constraint tangent L10 A2
  constraint tangent L9 A2
  constraint equal A0 A2
  constraint tangent L10 A3
  constraint tangent L11 A3
  constraint equal A0 A3
  measures "d115" radius of A0
sketch "Sketch37" plane through (0, 116.2145, -31.1396) normal (0, 0.965926, -0.258819) x (-1, 0, 0)
  ellipse E0 centre (22.741, -39.3535) end of major axis (22.741, -46.5838) minor radius 7 (22.741, -46.5838) -> (29.741, -39.3535) ccw
  line L0 (29.741, -39.3535) -> (29.741, 209.5755)
  ellipse E1 centre (22.741, 209.5755) end of major axis (22.741, 216.8058) minor radius 7 (29.741, 209.5755) -> (22.741, 216.8058) ccw
  line L1 (22.741, 216.8058) -> (-123.259, 216.8058)
  ellipse E2 centre (-123.259, 209.5755) end of major axis (-123.259, 216.8058) minor radius 7 (-123.259, 216.8058) -> (-130.259, 209.5755) ccw
  line L2 (-130.259, 209.5755) -> (-130.259, -39.3535)
  ellipse E3 centre (-123.259, -39.3535) end of major axis (-123.259, -46.5838) minor radius 7 (-130.259, -39.3535) -> (-123.259, -46.5838) ccw
  line L3 (-123.259, -46.5838) -> (22.741, -46.5838)
  line L4 (-35.9419, 179.9959) -> (-35.9419, 150.9959)
  line L5 (-35.9419, 150.9959) -> (-72.9419, 150.9959)
  line L6 (-72.9419, 150.9959) -> (-72.9419, 179.9959)
  line L7 (-72.9419, 179.9959) -> (-35.9419, 179.9959)
  line L8 (10, 30) -> (-10, 30)
  line L9 (-20, 40) -> (-20, 60)
  line L10 (-10, 70) -> (10, 70)
  line L11 (20, 60) -> (20, 40)
  line L12 (-40, 70) -> (-110, 70)
  line L13 (-120, 60) -> (-120, 40)
  line L14 (-110, 30) -> (-40, 30)
  line L15 (-30, 40) -> (-30, 60)
  arc A0 (-110, 70) -> (-120, 60) centre (-110, 60) ccw
  arc A1 (-30, 60) -> (-40, 70) centre (-40, 60) ccw
  arc A2 (-40, 30) -> (-30, 40) centre (-40, 40) ccw
  arc A3 (-120, 40) -> (-110, 30) centre (-110, 40) ccw
  arc A4 (-20, 40) -> (-10, 30) centre (-10, 40) ccw
  arc A5 (20, 60) -> (10, 70) centre (10, 60) ccw
  arc A6 (10, 30) -> (20, 40) centre (10, 40) ccw
  arc A7 (-10, 70) -> (-20, 60) centre (-10, 60) ccw
  dimension "d118" = 10
  constraint horizontal L8
  constraint vertical L9
  constraint horizontal L10
  constraint vertical L11
  constraint horizontal L12
  constraint vertical L13
  constraint horizontal L14
  constraint vertical L15
  constraint tangent L12 A0
  constraint tangent L13 A0
  constraint tangent L12 A1
  constraint tangent L15 A1
  constraint equal A0 A1
  constraint tangent L14 A2
  constraint tangent L15 A2
  constraint equal A0 A2
  constraint tangent L13 A3
  constraint tangent L14 A3
  constraint equal A0 A3
  constraint tangent L8 A4
  constraint tangent L9 A4
  constraint equal A0 A4
  constraint tangent L10 A5
  constraint tangent L11 A5
  constraint equal A0 A5
  constraint tangent L8 A6
  constraint tangent L11 A6
  constraint equal A0 A6
  constraint tangent L10 A7
  constraint tangent L9 A7
  constraint equal A0 A7
  measures "d118" radius of A0
sketch "Sketch38" plane through (0, 116.2145, -31.1396) normal (0, 0.965926, -0.258819) x (-1, 0, 0)
  line L0 (-40, 30) -> (-110, 30)
  arc A0 (-120, 40) -> (-110, 30) centre (-110, 40) ccw
  line L1 (-120, 40) -> (-120, 60)
  arc A1 (-110, 70) -> (-120, 60) centre (-110, 60) ccw
  line L2 (-110, 70) -> (-40, 70)
  arc A2 (-30, 60) -> (-40, 70) centre (-40, 60) ccw
  line L3 (-30, 60) -> (-30, 40)
  arc A3 (-40, 30) -> (-30, 40) centre (-40, 40) ccw
  line L4 (-10, 70) -> (10, 70)
  arc A4 (20, 60) -> (10, 70) centre (10, 60) ccw
  line L5 (20, 60) -> (20, 40)
  arc A5 (10, 30) -> (20, 40) centre (10, 40) ccw
  line L6 (10, 30) -> (-10, 30)
  arc A6 (-20, 40) -> (-10, 30) centre (-10, 40) ccw
  line L7 (-20, 40) -> (-20, 60)
  arc A7 (-10, 70) -> (-20, 60) centre (-10, 60) ccw
  ellipse E0 centre (22.741, -39.3535) end of major axis (22.741, -46.5838) minor radius 7 (22.741, -46.5838) -> (29.741, -39.3535) ccw
  line L8 (29.741, -39.3535) -> (29.741, 209.5755)
  ellipse E1 centre (22.741, 209.5755) end of major axis (22.741, 216.8058) minor radius 7 (29.741, 209.5755) -> (22.741, 216.8058) ccw
  line L9 (22.741, 216.8058) -> (-123.259, 216.8058)
  ellipse E2 centre (-123.259, 209.5755) end of major axis (-123.259, 216.8058) minor radius 7 (-123.259, 216.8058) -> (-130.259, 209.5755) ccw
  line L10 (-130.259, 209.5755) -> (-130.259, -39.3535)
  ellipse E3 centre (-123.259, -39.3535) end of major axis (-123.259, -46.5838) minor radius 7 (-130.259, -39.3535) -> (-123.259, -46.5838) ccw
  line L11 (-123.259, -46.5838) -> (22.741, -46.5838)
  line L12 (-35.9419, 179.9959) -> (-35.9419, 150.9959)
  line L13 (-35.9419, 150.9959) -> (-72.9419, 150.9959)
  line L14 (-72.9419, 150.9959) -> (-72.9419, 179.9959)
  line L15 (-72.9419, 179.9959) -> (-35.9419, 179.9959)
  line L16 (-110, 110) -> (-61.6636, 110)
  line L17 (-51.6636, 100) -> (-51.6636, 85)
  line L18 (-61.6636, 75) -> (-110, 75)
  line L19 (-120, 85) -> (-120, 100)
  line L20 (-35.44, 75) -> (-20, 75)
  line L21 (-10, 85) -> (-10, 100)
  line L22 (-20, 110) -> (-35.44, 110)
  line L23 (-45.44, 100) -> (-45.44, 85)
  line L24 (7.9281, 110) -> (12.9316, 110)
  line L25 (22.9316, 100) -> (22.9316, 85)
  line L26 (12.9316, 75) -> (7.9281, 75)
  line L27 (-2.0719, 85) -> (-2.0719, 100)
  arc A8 (-110, 110) -> (-120, 100) centre (-110, 100) ccw
  arc A9 (-51.6636, 100) -> (-61.6636, 110) centre (-61.6636, 100) ccw
  arc A10 (-61.6636, 75) -> (-51.6636, 85) centre (-61.6636, 85) ccw
  arc A11 (-120, 85) -> (-110, 75) centre (-110, 85) ccw
  arc A12 (-45.44, 85) -> (-35.44, 75) centre (-35.44, 85) ccw
  arc A13 (-10, 100) -> (-20, 110) centre (-20, 100) ccw
  arc A14 (-20, 75) -> (-10, 85) centre (-20, 85) ccw
  arc A15 (-35.44, 110) -> (-45.44, 100) centre (-35.44, 100) ccw
  arc A16 (7.9281, 110) -> (-2.0719, 100) centre (7.9281, 100) ccw
  arc A17 (12.9316, 75) -> (22.9316, 85) centre (12.9316, 85) ccw
  arc A18 (-2.0719, 85) -> (7.9281, 75) centre (7.9281, 85) ccw
  arc A19 (22.9316, 100) -> (12.9316, 110) centre (12.9316, 100) ccw
  dimension "d121" = 10
  constraint horizontal L16
  constraint vertical L17
  constraint horizontal L18
  constraint vertical L19
  constraint horizontal L20
  constraint vertical L21
  constraint horizontal L22
  constraint vertical L23
  constraint horizontal L24
  constraint vertical L25
  constraint horizontal L26
  constraint vertical L27
  constraint tangent L16 A8
  constraint tangent L19 A8
  constraint tangent L16 A9
  constraint tangent L17 A9
  constraint equal A8 A9
  constraint tangent L18 A10
  constraint tangent L17 A10
  constraint equal A8 A10
  constraint tangent L18 A11
  constraint tangent L19 A11
  constraint equal A8 A11
  constraint tangent L20 A12
  constraint tangent L23 A12
  constraint equal A8 A12
  constraint tangent L22 A13
  constraint tangent L21 A13
  constraint equal A8 A13
  constraint tangent L20 A14
  constraint tangent L21 A14
  constraint equal A8 A14
  constraint tangent L22 A15
  constraint tangent L23 A15
  constraint equal A8 A15
  constraint tangent L24 A16
  constraint tangent L27 A16
  constraint equal A8 A16
  constraint tangent L25 A17
  constraint tangent L26 A17
  constraint equal A8 A17
  constraint tangent L26 A18
  constraint tangent L27 A18
  constraint equal A8 A18
  constraint tangent L25 A19
  constraint tangent L24 A19
  constraint equal A8 A19
  measures "d121" radius of A8
sketch "Sketch39" plane through (0, 116.2145, -31.1396) normal (0, 0.965926, -0.258819) x (-1, 0, 0)
  line L0 (-120, 85) -> (-120, 100)
  arc A0 (-110, 110) -> (-120, 100) centre (-110, 100) ccw
  line L1 (-110, 110) -> (-61.6636, 110)
  arc A1 (-51.6636, 100) -> (-61.6636, 110) centre (-61.6636, 100) ccw
  line L2 (-51.6636, 100) -> (-51.6636, 85)
  arc A2 (-61.6636, 75) -> (-51.6636, 85) centre (-61.6636, 85) ccw
  line L3 (-61.6636, 75) -> (-110, 75)
  arc A3 (-120, 85) -> (-110, 75) centre (-110, 85) ccw
  line L4 (-45.44, 85) -> (-45.44, 100)
  arc A4 (-35.44, 110) -> (-45.44, 100) centre (-35.44, 100) ccw
  line L5 (-35.44, 110) -> (-20, 110)
  arc A5 (-10, 100) -> (-20, 110) centre (-20, 100) ccw
  line L6 (-10, 100) -> (-10, 85)
  arc A6 (-20, 75) -> (-10, 85) centre (-20, 85) ccw
  line L7 (-20, 75) -> (-35.44, 75)
  arc A7 (-45.44, 85) -> (-35.44, 75) centre (-35.44, 85) ccw
  line L8 (22.9316, 100) -> (22.9316, 85)
  arc A8 (12.9316, 75) -> (22.9316, 85) centre (12.9316, 85) ccw
  line L9 (12.9316, 75) -> (7.9281, 75)
  arc A9 (-2.0719, 85) -> (7.9281, 75) centre (7.9281, 85) ccw
  line L10 (-2.0719, 85) -> (-2.0719, 100)
  arc A10 (7.9281, 110) -> (-2.0719, 100) centre (7.9281, 100) ccw
  line L11 (7.9281, 110) -> (12.9316, 110)
  arc A11 (22.9316, 100) -> (12.9316, 110) centre (12.9316, 100) ccw
  line L12 (-40, 30) -> (-110, 30)
  arc A12 (-120, 40) -> (-110, 30) centre (-110, 40) ccw
  line L13 (-120, 40) -> (-120, 60)
  arc A13 (-110, 70) -> (-120, 60) centre (-110, 60) ccw
  line L14 (-110, 70) -> (-40, 70)
  arc A14 (-30, 60) -> (-40, 70) centre (-40, 60) ccw
  line L15 (-30, 60) -> (-30, 40)
  arc A15 (-40, 30) -> (-30, 40) centre (-40, 40) ccw
  line L16 (-10, 70) -> (10, 70)
  arc A16 (20, 60) -> (10, 70) centre (10, 60) ccw
  line L17 (20, 60) -> (20, 40)
  arc A17 (10, 30) -> (20, 40) centre (10, 40) ccw
  line L18 (10, 30) -> (-10, 30)
  arc A18 (-20, 40) -> (-10, 30) centre (-10, 40) ccw
  line L19 (-20, 40) -> (-20, 60)
  arc A19 (-10, 70) -> (-20, 60) centre (-10, 60) ccw
  ellipse E0 centre (22.741, -39.3535) end of major axis (22.741, -46.5838) minor radius 7 (22.741, -46.5838) -> (29.741, -39.3535) ccw
  line L20 (29.741, -39.3535) -> (29.741, 209.5755)
  ellipse E1 centre (22.741, 209.5755) end of major axis (22.741, 216.8058) minor radius 7 (29.741, 209.5755) -> (22.741, 216.8058) ccw
  line L21 (22.741, 216.8058) -> (-123.259, 216.8058)
  ellipse E2 centre (-123.259, 209.5755) end of major axis (-123.259, 216.8058) minor radius 7 (-123.259, 216.8058) -> (-130.259, 209.5755) ccw
  line L22 (-130.259, 209.5755) -> (-130.259, -39.3535)
  ellipse E3 centre (-123.259, -39.3535) end of major axis (-123.259, -46.5838) minor radius 7 (-130.259, -39.3535) -> (-123.259, -46.5838) ccw
  line L23 (-123.259, -46.5838) -> (22.741, -46.5838)
  line L24 (-35.9419, 179.9959) -> (-35.9419, 150.9959)
  line L25 (-35.9419, 150.9959) -> (-72.9419, 150.9959)
  line L26 (-72.9419, 150.9959) -> (-72.9419, 179.9959)
  line L27 (-72.9419, 179.9959) -> (-35.9419, 179.9959)
  line L28 (-109.8689, 117.075) -> (-111.5449, 117.075)
  line L29 (-116.5449, 122.075) -> (-116.5449, 197.0502)
  line L30 (-111.5449, 202.0502) -> (-109.8689, 202.0502)
  line L31 (-104.8689, 197.0502) -> (-104.8689, 122.075)
  line L32 (-95.6526, 202.0502) -> (-95.5983, 202.0502)
  line L33 (-90.5983, 197.0502) -> (-90.5983, 159.5626)
  line L34 (-90.5983, 159.5626) -> (-100.6526, 159.5626)
  line L35 (-100.6526, 159.5626) -> (-100.6526, 197.0502)
  line L36 (-100.6526, 154.3733) -> (-90.5983, 154.3733)
  line L37 (-90.5983, 154.3733) -> (-90.5983, 122.0948)
  line L38 (-95.5983, 117.0948) -> (-95.6526, 117.0948)
  line L39 (-100.6526, 122.0948) -> (-100.6526, 154.3733)
  line L40 (-79.2974, 201.948) -> (-81.4093, 201.948)
  line L41 (-76.4093, 196.948) -> (-76.4093, 176.5782)
  line L42 (-76.4093, 176.5782) -> (-84.2974, 176.5782)
  line L43 (-84.2974, 176.5782) -> (-84.2974, 196.948)
  line L44 (-84.2974, 171.0352) -> (-76.4093, 171.0352)
  line L45 (-76.4093, 171.0352) -> (-76.4093, 121.8844)
  line L46 (-81.4093, 116.8844) -> (-79.2974, 116.8844)
  line L47 (-84.2974, 121.8844) -> (-84.2974, 171.0352)
  line L48 (-67.5, 145) -> (-37.5, 145)
  line L49 (-35, 142.5) -> (-35, 137.5)
  line L50 (-37.5, 135) -> (-67.5, 135)
  line L51 (-70, 137.5) -> (-70, 142.5)
  line L52 (-65, 130) -> (-40, 130)
  line L53 (-35, 125) -> (-35, 117.5)
  line L54 (-37.5, 115) -> (-65, 115)
  line L55 (-70, 120) -> (-70, 125)
  arc A20 (-67.5, 145) -> (-70, 142.5) centre (-67.5, 142.5) ccw
  arc A21 (-70, 137.5) -> (-67.5, 135) centre (-67.5, 137.5) ccw
  arc A22 (-35, 142.5) -> (-37.5, 145) centre (-37.5, 142.5) ccw
  arc A23 (-37.5, 135) -> (-35, 137.5) centre (-37.5, 137.5) ccw
  arc A24 (-35, 127.5) -> (-37.5, 130) centre (-37.5, 127.5) ccw
  arc A25 (-37.5, 115) -> (-35, 117.5) centre (-37.5, 117.5) ccw
  arc A26 (-70, 120) -> (-65, 115) centre (-65, 120) ccw
  arc A27 (-65, 130) -> (-70, 125) centre (-65, 125) ccw
  arc A28 (-35, 125) -> (-40, 130) centre (-40, 125) ccw
  arc A29 (-111.5449, 202.0502) -> (-116.5449, 197.0502) centre (-111.5449, 197.0502) ccw
  arc A30 (-104.8689, 197.0502) -> (-109.8689, 202.0502) centre (-109.8689, 197.0502) ccw
  arc A31 (-95.6526, 202.0502) -> (-100.6526, 197.0502) centre (-95.6526, 197.0502) ccw
  arc A32 (-90.5983, 197.0502) -> (-95.5983, 202.0502) centre (-95.5983, 197.0502) ccw
  arc A33 (-79.2974, 201.948) -> (-84.2974, 196.948) centre (-79.2974, 196.948) ccw
  arc A34 (-76.4093, 196.948) -> (-81.4093, 201.948) centre (-81.4093, 196.948) ccw
  arc A35 (-116.5449, 122.075) -> (-111.5449, 117.075) centre (-111.5449, 122.075) ccw
  arc A36 (-109.8689, 117.075) -> (-104.8689, 122.075) centre (-109.8689, 122.075) ccw
  arc A37 (-100.6526, 122.0948) -> (-95.6526, 117.0948) centre (-95.6526, 122.0948) ccw
  arc A38 (-95.5983, 117.0948) -> (-90.5983, 122.0948) centre (-95.5983, 122.0948) ccw
  arc A39 (-84.2974, 121.8844) -> (-79.2974, 116.8844) centre (-79.2974, 121.8844) ccw
  arc A40 (-81.4093, 116.8844) -> (-76.4093, 121.8844) centre (-81.4093, 121.8844) ccw
  dimension "d124" = 2.5
  dimension "d125" = 5
  constraint horizontal L28
  constraint vertical L29
  constraint horizontal L30
  constraint vertical L31
  constraint horizontal L32
  constraint vertical L33
  constraint horizontal L34
  constraint vertical L35
  constraint horizontal L36
  constraint vertical L37
  constraint horizontal L38
  constraint vertical L39
  constraint horizontal L40
  constraint vertical L41
  constraint horizontal L42
  constraint vertical L43
  constraint horizontal L44
  constraint vertical L45
  constraint horizontal L46
  constraint vertical L47
  constraint horizontal L48
  constraint vertical L49
  constraint horizontal L50
  constraint vertical L51
  constraint horizontal L52
  constraint vertical L53
  constraint horizontal L54
  constraint vertical L55
  constraint tangent L48 A20
  constraint tangent L51 A20
  constraint tangent L50 A21
  constraint tangent L51 A21
  constraint equal A20 A21
  constraint tangent L48 A22
  constraint tangent L49 A22
  constraint equal A20 A22
  constraint tangent L49 A23
  constraint tangent L50 A23
  constraint equal A20 A23
  constraint tangent L52 A24
  constraint tangent L53 A24
  constraint equal A20 A24
  constraint tangent L53 A25
  constraint tangent L54 A25
  constraint equal A20 A25
  constraint tangent L54 A26
  constraint tangent L55 A26
  constraint tangent L52 A27
  constraint tangent L55 A27
  constraint equal A26 A27
  constraint coincident L52 A24.end
  constraint coincident L53 A24.start
  constraint tangent L52 A28
  constraint tangent L53 A28
  constraint equal A26 A28
  constraint tangent L29 A29
  constraint tangent L30 A29
  constraint equal A26 A29
  constraint tangent L30 A30
  constraint tangent L31 A30
  constraint equal A26 A30
  constraint tangent L32 A31
  constraint tangent L35 A31
  constraint equal A26 A31
  constraint tangent L32 A32
  constraint tangent L33 A32
  constraint equal A26 A32
  constraint tangent L40 A33
  constraint tangent L43 A33
  constraint equal A26 A33
  constraint tangent L40 A34
  constraint tangent L41 A34
  constraint equal A26 A34
  constraint tangent L28 A35
  constraint tangent L29 A35
  constraint equal A26 A35
  constraint tangent L28 A36
  constraint tangent L31 A36
  constraint equal A26 A36
  constraint tangent L38 A37
  constraint tangent L39 A37
  constraint equal A26 A37
  constraint tangent L37 A38
  constraint tangent L38 A38
  constraint equal A26 A38
  constraint tangent L46 A39
  constraint tangent L47 A39
  constraint equal A26 A39
  constraint tangent L45 A40
  constraint tangent L46 A40
  constraint equal A26 A40
  measures "d124" radius of A20
  measures "d125" radius of A26